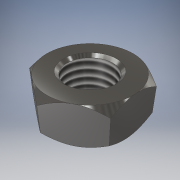
# Autodesk Inventor part: Nut-M3
Saved by Autodesk Inventor 2018 (Build 220112000, 112)
## iProperties
Created: 2020-04-17
Part Number: Nut-M3
Material: Ocel, vysokopevnostní, nízkolegovaná
Document SubType Name: Modeling
Designer: Jozko Mrkvicka
Density: 7.85 g/cm^3
Appearance: Ocel – leštěná
Author: Jozko Mrkvicka
Autodesk Inventor part; units mm, degrees
ref_plane "YZ Plane" through (0, 0, 0) normal (1, 0, 0) x (0, 1, 0)
ref_plane "XZ Plane" through (0, 0, 0) normal (0, 1, 0) x (-1, 0, 0)
ref_plane "XY Plane" through (0, 0, 0) normal (0, 0, 1) x (1, 0, 0)
sketch "Náčrt1" plane through (0, 0, 0) normal (0, 0, 1) x (1, 0, 0)
  line L0 (2.75, -1.5877) -> (0, -3.1754)
  line L1 (0, -3.1754) -> (-2.75, -1.5877)
  line L2 (-2.75, -1.5877) -> (-2.75, 1.5877)
  line L3 (-2.75, 1.5877) -> (0, 3.1754)
  line L4 (0, 3.1754) -> (2.75, 1.5877)
  line L5 (2.75, 1.5877) -> (2.75, -1.5877)
  circle A0 centre (0, 0) radius 1.5
  point P0 (2.75, 0)
  dimension "d1" = 3
  constraints: 12 end point, 1 centre point, 1 coincident, 1 midpoint, 13 other
  measures "d1" diameter of A0
extrude "Vysunutí1" add sketch "Náčrt1" along normal blind 2.4
thread "Závit1" size "M3x0.5" class "6H" standard "ANSI Metric M Profile" full length
sketch "Náčrt2" plane through (0, 0, 2.4) normal (0, 0, 1) x (1, 0, 0)
  circle A0 centre (0, 0) radius 2.75
  constraints: 1 centre point, 1 coincident
extrude "Vysunutí2" cut sketch "Náčrt2" against normal through all draft 45 keep common part
sketch "Náčrt3" plane through (0, 0, 0) normal (0, 0, -1) x (-1, 0, 0)
  circle A0 centre (0, 0) radius 2.75
  constraints: 1 centre point, 1 coincident
extrude "Vysunutí3" cut sketch "Náčrt3" against normal through all draft 45 keep common part
chamfer "Zkosení1" distance 0.2 angle 45 1 edges at (-1.5, 0, 2.4)
chamfer "Zkosení2" distance 0.2 angle 45 1 edges at (-1.5, 0, 0)
